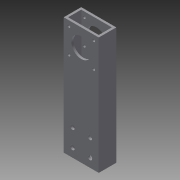
# Autodesk Inventor part: Z-Bar
Saved by Autodesk Inventor 2013 (Build 170138000, 138)
## iProperties
Created: 2014-01-24
Part Number: Z-Bar
Material: Generic
Document SubType Name: Modeling
Designer: Jarod
Density: 1 g/cm^3
Author: Jarod
Autodesk Inventor part; units mm, degrees
ref_plane "YZ Plane" through (0, 0, 0) normal (1, 0, 0) x (0, 1, 0)
ref_plane "XZ Plane" through (0, 0, 0) normal (0, 1, 0) x (-1, 0, 0)
ref_plane "XY Plane" through (0, 0, 0) normal (0, 0, 1) x (1, 0, 0)
sketch "Sketch1" plane through (0, 0, 0) normal (0, 0, 1) x (1, 0, 0)
  line L0 (0, 0) -> (50.8, 0)
  line L1 (50.8, 0) -> (50.8, 169.8752)
  line L2 (50.8, 169.8752) -> (0, 169.8752)
  line L3 (0, 169.8752) -> (0, 0)
  line L4 (25.4, 169.8752) -> (25.4, 144.4752)
  line L5 (25.4, 169.8752) -> (50.8, 169.8752) construction
  circle A0 centre (25.4, 144.4752) radius 14.2875
  line L6 (25.4, 144.4752) -> (43.3605, 162.4357)
  line L7 (25.4, 144.4752) -> (50.8, 144.4752) construction
  line L8 (7.4395, 126.5147) -> (43.3605, 126.5147)
  line L9 (43.3605, 162.4357) -> (7.4395, 162.4357)
  line L10 (7.4395, 162.4357) -> (7.4395, 126.5147)
  circle A1 centre (7.4395, 162.4357) radius 2.032
  circle A2 centre (7.4395, 126.5147) radius 2.032
  circle A3 centre (43.3605, 162.4357) radius 2.032
  circle A4 centre (43.3605, 126.5147) radius 2.032
  line L11 (0, 0) -> (50.8, 0)
  line L12 (50.8, 0) -> (50.8, 38.1)
  line L13 (0, 38.1) -> (0, 0)
  line L14 (25.4, 38.1) -> (12.7, 38.1)
  line L15 (25.4, 38.1) -> (38.1, 38.1) construction
  line L16 (12.7, 38.1) -> (38.1, 38.1)
  circle A5 centre (12.7, 38.1) radius 3.175
  circle A6 centre (38.1, 38.1) radius 3.175
  dimension "d0" = 50.8
  dimension "d1" = 169.8752
  dimension "d2" = 25.4
  dimension "d3" = 90
  dimension "d4" = 28.575
  dimension "d5" = 25.4
  dimension "d6" = 45
  dimension "d7" = 50.8
  dimension "d9" = 4.064
  dimension "d10" = 4.064
  dimension "d11" = 4.064
  dimension "d12" = 4.064
  dimension "d13" = 50.8
  dimension "d14" = 38.1
  dimension "d15" = 12.7
  dimension "d16" = 180
  dimension "d17" = 25.4
  dimension "d18" = 0
  dimension "d19" = 6.35
  dimension "d20" = 6.35
  constraints: 34 end point, 7 centre point, 7 coincident, 6 horizontal, 5 parallel, 3 equal length, 2 perpendicular, 1 midpoint
  measures "d0" distance of L2.end L1.end
  measures "d1" distance of L1.end L0.end
  measures "d2" distance of L4.start L4.end
  measures "d3" angle of L4 L5
  measures "d4" diameter of A0
  measures "d5" distance of L6.start L6.end
  measures "d6" angle of L7 L6
  measures "d7" distance of L6.end L8.start
  measures "d9" diameter of A1
  measures "d10" diameter of A2
  measures "d11" diameter of A3
  measures "d12" diameter of A4
  measures "d13" distance of L13.start L12.end
  measures "d14" distance of L12.end L11.end
  measures "d15" distance of L14.start L14.end
  measures "d16" angle of L14 L15
  measures "d17" distance of L14.end L16.end
  measures "d18" distance between parallel lines of L16 L14
  measures "d19" diameter of A5
  measures "d20" diameter of A6
extrude "Extrusion1" add sketch "Sketch1" along normal blind 25.4 contours L3 L2 L1 L0 | L9 A3 L6 A0 L4
sketch "Sketch2" plane through (0, 169.8752, 0) normal (0, 1, 0) x (1, 0, 0)
  line L0 (0, 0) -> (3.175, 0)
  line L1 (3.175, 0) -> (3.175, -3.175)
  line L2 (3.175, -3.175) -> (0, -3.175)
  line L3 (0, -3.175) -> (0, 0)
  line L4 (3.175, -3.175) -> (47.625, -3.175)
  line L5 (47.625, -3.175) -> (47.625, -22.225)
  line L6 (47.625, -22.225) -> (3.175, -22.225)
  line L7 (3.175, -22.225) -> (3.175, -3.175)
  dimension "d23" = 3.175
  dimension "d24" = 3.175
  dimension "d25" = 44.45
  dimension "d26" = 19.05
  constraints: 16 end point, 4 parallel, 2 horizontal, 2 perpendicular
  measures "d23" distance of L1.end L2.end
  measures "d24" distance of L0.end L1.end
  measures "d25" distance of L5.end L6.end
  measures "d26" distance of L4.end L5.end
extrude "Extrusion2" cut sketch "Sketch2" against normal blind 254 contours L4 L5 L6 L7
sketch "Sketch3" plane through (0, 0, 25.4) normal (0, 0, 1) x (1, 0, 0)
  circle A0 centre (12.7, 38.1) radius 3.175 projected
  line L0 (12.7, 38.1) -> (38.1, 38.1)
  line L1 (38.1, 38.1) -> (38.1, 12.7)
  line L2 (38.1, 12.7) -> (12.7, 12.7)
  line L3 (12.7, 12.7) -> (12.7, 38.1)
  circle A1 centre (12.7, 12.7) radius 3.175
  circle A2 centre (38.1, 12.7) radius 3.175
  dimension "d29" = 25.4
  dimension "d30" = 25.4
  dimension "d31" = 6.35
  dimension "d32" = 6.35
  constraints: 8 end point, 2 centre point, 2 coincident, 2 parallel, 1 horizontal, 1 perpendicular
  measures "d29" distance of L1.end L2.end
  measures "d30" distance of L0.end L1.end
  measures "d31" diameter of A1
  measures "d32" diameter of A2
extrude "Extrusion3" cut sketch "Sketch3" against normal blind 25.4 contours A1 L2 L3 | L3 L2 A1 | A2 L2 L1 | L1 L2 A2
body "Solid1"
